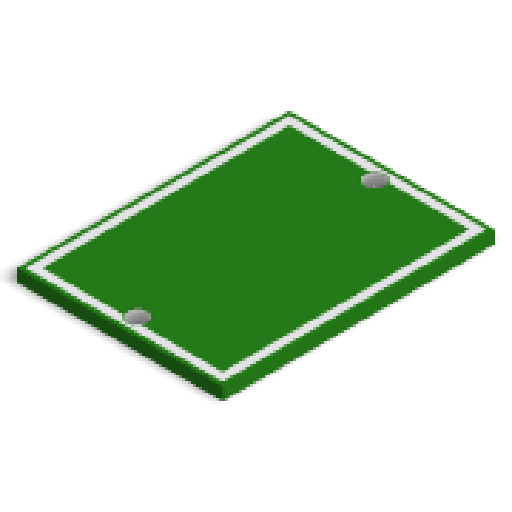
# Autodesk Inventor part: PIR sensor
Saved by Autodesk Inventor 2024 (Build 280153000, 153)
## iProperties
Created: 2024-09-23
Part Number: PIR sensor
Material: Generic
Document SubType Name: Modeling
Designer: Laith Al-Sadi
Density: 1 g/cm^3
Appearance: Default
Author: Laith Al-Sadi
Autodesk Inventor part; units mm, degrees
ref_plane "YZ Plane" through (0, 0, 0) normal (1, 0, 0) x (0, 1, 0)
ref_plane "XZ Plane" through (0, 0, 0) normal (0, 1, 0) x (-1, 0, 0)
ref_plane "XY Plane" through (0, 0, 0) normal (0, 0, 1) x (1, 0, 0)
sketch "Sketch1" plane through (0, 0, 0) normal (0, 1, 0) x (-1, 0, 0)
  line L0 (12.15, 16.1) -> (-12.15, 16.1)
  line L1 (-12.15, 16.1) -> (-12.15, -16.1)
  line L2 (-12.15, -16.1) -> (12.15, -16.1)
  line L3 (12.15, -16.1) -> (12.15, 16.1)
  line L4 (12.15, 16.1) -> (-12.15, -16.1) construction
  line L5 (-12.15, 16.1) -> (12.15, -16.1) construction
  circle A0 centre (0, 14) radius 1.15
  circle A1 centre (0, -14) radius 1.15
  point P0 (0, 0)
  dimension "d0" = 32.2
  dimension "d1" = 24.3
  dimension "d4" = 2.3
  dimension "d5" = 2.3
  dimension "d6" = 28
  dimension "d7" = 14
  constraints: 12 end point, 2 centre point, 2 midpoint, 2 parallel, 2 vertical alignment, 1 horizontal, 1 perpendicular
  measures "d0" distance of L2.end L0.start
  measures "d1" distance of L1.end L2.end
  measures "d4" diameter of A0
  measures "d5" diameter of A1
  measures "d6" distance of A1.centre A0.centre
  measures "d7" distance of point (0, 0) A0.centre
extrude "Extrusion1" add sketch "Sketch1" along normal blind 1.5
sketch "Sketch2" plane through (0, 1.5, 0) normal (0, 1, 0) x (1, 0, 0)
  line L0 (12.15, -16.1) -> (12.15, 16.1) projected
  line L1 (12.15, 16.1) -> (-12.15, 16.1) projected
  line L2 (-12.15, 16.1) -> (-12.15, -16.1) projected
  line L3 (-12.15, -16.1) -> (12.15, -16.1) projected
  circle A0 centre (0, -14) radius 1.15 projected
  circle A1 centre (0, 14) radius 1.15 projected
  line L4 (-11.65, -15.6) -> (-11.65, 15.6)
  line L5 (-11.65, 15.6) -> (11.65, 15.6)
  line L6 (11.65, 15.6) -> (11.65, -15.6)
  line L7 (11.65, -15.6) -> (-11.65, -15.6)
  line L8 (-10.65, 14.6) -> (-10.65, -14.6)
  line L9 (-10.65, -14.6) -> (10.65, -14.6)
  line L10 (10.65, -14.6) -> (10.65, 14.6)
  line L11 (10.65, 14.6) -> (-10.65, 14.6)
  point P0 (0, 0)
  point P1 (-0.9811, 14.6)
  point P2 (0.9811, 14.6)
  point P3 (0.9811, -14.6)
  point P4 (-0.9811, -14.6)
  dimension "d8" = 0.5
  dimension "d9" = 1
  constraints: 16 end point, 6 other
  measures "d8" distance between parallel lines of L2 L4
  measures "d9" distance between parallel lines of L4 L8
extrude "Extrusion2" add sketch "Sketch2" along normal blind 0.01 contours L4 L5 L6 L7
sketch "Sketch3" plane through (0, 1.5, 0) normal (0, 1, 0) x (1, 0, 0)
  circle A0 centre (0, -14) radius 1.15 projected
  circle A1 centre (0, -14) radius 1.2525
  arc A2 (-0.9811, 14.6) -> (0.9811, 14.6) centre (0, 14) ccw projected
  circle A3 centre (0, 14) radius 1.2525
  point P0 (0, 0)
  dimension "d12" = 2.505
  dimension "d13" = 2.505
  constraints: 2 centre point, 2 coincident
  measures "d12" diameter of A1
  measures "d13" diameter of A3
extrude "Extrusion3" cut sketch "Sketch3" along normal up to surface (0.01 mm away)
sketch "Sketch4" plane through (0, 0, 0) normal (0, -1, 0) x (1, 0, 0)
  line L0 (-11.45, 3) -> (-11.45, -3) construction
  line L1 (-11.45, -3) -> (-12.15, -3) construction
  line L2 (-12.15, -3) -> (-12.15, 3) construction
  line L3 (-12.15, 3) -> (-11.45, 3) construction
  line L4 (-12.15, -16.1) -> (-12.15, 16.1) projected
  line L5 (11.3793, -5.3256) -> (11.3793, 5.3256) construction
  line L6 (11.3793, 5.3256) -> (20.3774, 5.3256) construction
  line L7 (20.3774, 5.3256) -> (20.3774, -5.3256) construction
  line L8 (20.3774, -5.3256) -> (11.3793, -5.3256) construction
  line L9 (12.15, 16.1) -> (12.15, -16.1) projected
  spline S0 degree 2 poles (-11.6479, 2.8207) (-11.7346, 2.8207) (-11.8493, 2.7865) (-11.8493, 2.7444) knots 0 0 0 1 2 2 2
  spline S1 degree 2 poles (-11.8493, 2.7444) (-11.8493, 2.7237) (-11.8327, 2.7016) (-11.8127, 2.696) (-11.7851, 2.695) (-11.7647, 2.695) knots 0 0 0 1 2 3 4 4 4
  line L10 (-11.7647, 2.695) -> (-11.7433, 2.695)
  spline S2 degree 2 poles (-11.7433, 2.695) (-11.7198, 2.695) (-11.7115, 2.6967) knots 0 0 0 1 1 1
  spline S3 degree 2 poles (-11.7115, 2.6967) (-11.6935, 2.6981) (-11.6804, 2.7098) (-11.6769, 2.734) (-11.6766, 2.7537) (-11.6759, 2.762) knots 0 0 0 1 2 3 4 4 4
  line L11 (-11.6759, 2.762) -> (-11.6673, 2.762)
  line L12 (-11.6673, 2.762) -> (-11.6673, 2.505)
  line L13 (-11.6673, 2.505) -> (-11.6759, 2.505)
  line L14 (-11.6759, 2.505) -> (-11.6776, 2.5302)
  spline S4 degree 2 poles (-11.6776, 2.5302) (-11.6794, 2.5472) (-11.6918, 2.5585) (-11.7104, 2.5603) knots 0 0 0 1 2 2 2
  line L15 (-11.7104, 2.5603) -> (-11.7364, 2.5613)
  line L16 (-11.7364, 2.5613) -> (-11.8082, 2.5613)
  line L17 (-11.8082, 2.5613) -> (-11.8576, 2.5603)
  line L18 (-11.8576, 2.5603) -> (-11.8576, 2.5686)
  spline S5 degree 2 poles (-11.8576, 2.5686) (-11.8417, 2.5758) (-11.8151, 2.6114) (-11.8151, 2.6328) knots 0 0 0 1 2 2 2
  spline S6 degree 2 poles (-11.8151, 2.6328) (-11.8151, 2.6518) (-11.8624, 2.7233) (-11.8624, 2.782) knots 0 0 0 1 2 2 2
  spline S7 degree 2 poles (-11.8624, 2.782) (-11.8624, 2.8632) (-11.745, 2.9741) (-11.6562, 2.9741) knots 0 0 0 1 2 2 2
  spline S8 degree 2 poles (-11.6562, 2.9741) (-11.563, 2.9741) (-11.45, 2.8522) (-11.45, 2.7579) knots 0 0 0 1 2 2 2
  spline S9 degree 2 poles (-11.45, 2.7579) (-11.45, 2.7064) (-11.4959, 2.6142) (-11.497, 2.6086) knots 0 0 0 1 2 2 2
  spline S10 degree 2 poles (-11.497, 2.6086) (-11.497, 2.5927) (-11.4735, 2.5817) (-11.4514, 2.5769) knots 0 0 0 1 2 2 2
  line L19 (-11.4514, 2.5769) -> (-11.4514, 2.5658)
  line L20 (-11.4514, 2.5658) -> (-11.6286, 2.5658)
  line L21 (-11.6286, 2.5658) -> (-11.6286, 2.5751)
  spline S11 degree 2 poles (-11.6286, 2.5751) (-11.5609, 2.5917) (-11.4666, 2.668) (-11.4666, 2.7275) knots 0 0 0 1 2 2 2
  spline S12 degree 2 poles (-11.4666, 2.7275) (-11.4666, 2.7744) (-11.5757, 2.8207) (-11.6479, 2.8207) knots 0 0 0 1 2 2 2
  spline S13 degree 2 poles (-11.4645, 2.0093) (-11.4652, 2.0166) (-11.4662, 2.0335) (-11.4711, 2.0642) (-11.4915, 2.0801) (-11.5091, 2.0819) knots 0 0 0 1 2 3 4 4 4
  line L22 (-11.5091, 2.0819) -> (-11.5353, 2.0829)
  line L23 (-11.5353, 2.0829) -> (-11.8559, 2.0829)
  line L24 (-11.8559, 2.0829) -> (-11.8559, 2.1499)
  line L25 (-11.8559, 2.1499) -> (-11.5222, 2.4107)
  line L26 (-11.5222, 2.4107) -> (-11.5222, 2.4128)
  line L27 (-11.5222, 2.4128) -> (-11.7785, 2.4128)
  line L28 (-11.7785, 2.4128) -> (-11.8051, 2.4117)
  spline S14 degree 2 poles (-11.8051, 2.4117) (-11.8231, 2.41) (-11.8407, 2.3952) (-11.8455, 2.3651) (-11.8465, 2.3437) (-11.8472, 2.3399) knots 0 0 0 1 2 3 4 4 4
  line L29 (-11.8472, 2.3399) -> (-11.8559, 2.3399)
  line L30 (-11.8559, 2.3399) -> (-11.8559, 2.4981)
  line L31 (-11.8559, 2.4981) -> (-11.8472, 2.4981)
  spline S15 degree 2 poles (-11.8472, 2.4981) (-11.8465, 2.4908) (-11.8455, 2.4732) (-11.8386, 2.4287) (-11.8051, 2.4252) knots 0 0 0 1 2 3 3 3
  line L32 (-11.8051, 2.4252) -> (-11.7785, 2.4242)
  line L33 (-11.7785, 2.4242) -> (-11.5288, 2.4242)
  line L34 (-11.5288, 2.4242) -> (-11.5035, 2.4252)
  spline S16 degree 2 poles (-11.5035, 2.4252) (-11.4918, 2.4325) (-11.4721, 2.4522) (-11.4645, 2.476) (-11.4645, 2.487) knots 0 0 0 1 2 3 3 3
  line L35 (-11.4645, 2.487) -> (-11.4645, 2.5036)
  line L36 (-11.4645, 2.5036) -> (-11.4559, 2.5036)
  line L37 (-11.4559, 2.5036) -> (-11.4559, 2.2936)
  line L38 (-11.4559, 2.2936) -> (-11.7084, 2.0964)
  line L39 (-11.7084, 2.0964) -> (-11.7084, 2.0943)
  line L40 (-11.7084, 2.0943) -> (-11.5332, 2.0943)
  line L41 (-11.5332, 2.0943) -> (-11.507, 2.0953)
  spline S17 degree 2 poles (-11.507, 2.0953) (-11.4894, 2.0971) (-11.4711, 2.1119) (-11.4662, 2.1416) (-11.4652, 2.1596) (-11.4645, 2.1672) knots 0 0 0 1 2 3 4 4 4
  line L42 (-11.4645, 2.1672) -> (-11.4559, 2.1672)
  line L43 (-11.4559, 2.1672) -> (-11.4559, 2.0093)
  line L44 (-11.4559, 2.0093) -> (-11.4645, 2.0093)
  line L45 (-11.8559, 1.9921) -> (-11.8472, 1.9921)
  spline S18 degree 2 poles (-11.8472, 1.9921) (-11.8472, 1.9851) (-11.8455, 1.9665) (-11.8427, 1.9427) (-11.8293, 1.9302) (-11.8117, 1.9285) knots 0 0 0 1 2 3 4 4 4
  line L46 (-11.8117, 1.9285) -> (-11.7864, 1.9275)
  line L47 (-11.7864, 1.9275) -> (-11.526, 1.9275)
  line L48 (-11.526, 1.9275) -> (-11.5008, 1.9285)
  spline S19 degree 2 poles (-11.5008, 1.9285) (-11.4832, 1.9302) (-11.469, 1.9434) (-11.4655, 1.9668) (-11.4652, 1.9862) (-11.4645, 1.9938) knots 0 0 0 1 2 3 4 4 4
  line L49 (-11.4645, 1.9938) -> (-11.4559, 1.9938)
  line L50 (-11.4559, 1.9938) -> (-11.4545, 1.7893)
  spline S20 degree 2 poles (-11.4545, 1.7893) (-11.4545, 1.725) (-11.4787, 1.6114) (-11.5775, 1.5154) (-11.6676, 1.5154) knots 0 0 0 1 2 3 3 3
  spline S21 degree 2 poles (-11.6676, 1.5154) (-11.7536, 1.5154) (-11.8355, 1.6014) (-11.8559, 1.6974) (-11.8559, 1.7613) knots 0 0 0 1 2 3 3 3
  line L51 (-11.8559, 1.7613) -> (-11.8559, 1.9921)
  spline S22 degree 2 poles (-11.4718, 1.7344) (-11.4683, 1.7423) (-11.4662, 1.7744) (-11.4662, 1.7862) knots 0 0 0 1 2 2 2
  line L52 (-11.4662, 1.7862) -> (-11.4662, 1.7927)
  line L53 (-11.4662, 1.7927) -> (-11.8455, 1.7927)
  spline S23 degree 2 poles (-11.8455, 1.7927) (-11.8455, 1.7889) (-11.8462, 1.7824) (-11.8462, 1.7772) knots 0 0 0 1 2 2 2
  spline S24 degree 2 poles (-11.8462, 1.7772) (-11.8462, 1.7565) (-11.8407, 1.7219) (-11.8182, 1.6915) (-11.7212, 1.6636) (-11.67, 1.6636) knots 0 0 0 1 2 3 4 4 4
  spline S25 degree 2 poles (-11.67, 1.6636) (-11.5985, 1.6636) (-11.4859, 1.6981) (-11.4718, 1.7344) knots 0 0 0 1 2 2 2
  spline S26 degree 2 poles (-11.6562, 0.3344) (-11.744, 0.3344) (-11.8624, 0.4674) (-11.8624, 0.5579) knots 0 0 0 1 2 2 2
  spline S27 degree 2 poles (-11.8624, 0.5579) (-11.8624, 0.6522) (-11.7457, 0.7789) (-11.6562, 0.7789) knots 0 0 0 1 2 2 2
  spline S28 degree 2 poles (-11.6562, 0.7789) (-11.564, 0.7789) (-11.45, 0.6494) (-11.45, 0.5579) knots 0 0 0 1 2 2 2
  spline S29 degree 2 poles (-11.45, 0.5579) (-11.45, 0.466) (-11.5657, 0.3344) (-11.6562, 0.3344) knots 0 0 0 1 2 2 2
  spline S30 degree 2 poles (-11.5063, 0.5012) (-11.4604, 0.5174) (-11.4604, 0.5575) knots 0 0 0 1 1 1
  spline S31 degree 2 poles (-11.4604, 0.5575) (-11.4604, 0.5779) (-11.4866, 0.6076) (-11.5367, 0.6235) (-11.6151, 0.6307) (-11.6562, 0.6307) knots 0 0 0 1 2 3 4 4 4
  spline S32 degree 2 poles (-11.6562, 0.6307) (-11.7129, 0.6307) (-11.784, 0.6221) (-11.8521, 0.5979) (-11.8521, 0.5575) knots 0 0 0 1 2 3 3 3
  spline S33 degree 2 poles (-11.8521, 0.5575) (-11.8521, 0.5375) (-11.8258, 0.5078) (-11.7757, 0.4919) (-11.6973, 0.4846) (-11.6562, 0.4846) knots 0 0 0 1 2 3 4 4 4
  spline S34 degree 2 poles (-11.6562, 0.4846) (-11.6075, 0.4846) (-11.5357, 0.4912) (-11.5063, 0.5012) knots 0 0 0 1 2 2 2
  spline S35 degree 2 poles (-11.4645, -0.1689) (-11.4652, -0.1617) (-11.4662, -0.1434) (-11.4704, -0.1133) (-11.4925, -0.0974) (-11.5101, -0.0957) knots 0 0 0 1 2 3 4 4 4
  line L54 (-11.5101, -0.0957) -> (-11.5364, -0.0946)
  line L55 (-11.5364, -0.0946) -> (-11.6994, -0.0946)
  line L56 (-11.6994, -0.0946) -> (-11.727, -0.0936)
  spline S36 degree 2 poles (-11.727, -0.0936) (-11.8027, -0.0853) (-11.8624, -0.0193) (-11.8624, 0.0497) knots 0 0 0 1 2 2 2
  spline S37 degree 2 poles (-11.8624, 0.0497) (-11.8624, 0.1406) (-11.7934, 0.2394) (-11.7415, 0.2394) knots 0 0 0 1 2 2 2
  line L57 (-11.7415, 0.2394) -> (-11.5253, 0.2394)
  line L58 (-11.5253, 0.2394) -> (-11.5001, 0.2404)
  spline S38 degree 2 poles (-11.5001, 0.2404) (-11.4825, 0.2421) (-11.469, 0.2535) (-11.4666, 0.2708) knots 0 0 0 1 2 2 2
  line L59 (-11.4666, 0.2708) -> (-11.4645, 0.2936)
  line L60 (-11.4645, 0.2936) -> (-11.4559, 0.2936)
  line L61 (-11.4559, 0.2936) -> (-11.4559, 0.037)
  line L62 (-11.4559, 0.037) -> (-11.4645, 0.037)
  spline S39 degree 2 poles (-11.4645, 0.037) (-11.4652, 0.0442) (-11.4655, 0.0625) (-11.4693, 0.0908) (-11.4814, 0.1019) (-11.5001, 0.1036) knots 0 0 0 1 2 3 4 4 4
  line L63 (-11.5001, 0.1036) -> (-11.5256, 0.1047)
  line L64 (-11.5256, 0.1047) -> (-11.7457, 0.1047)
  spline S40 degree 2 poles (-11.7457, 0.1047) (-11.7522, 0.1047) (-11.7709, 0.1036) (-11.8099, 0.0974) (-11.8479, 0.0598) (-11.8479, 0.0266) knots 0 0 0 1 2 3 4 4 4
  spline S41 degree 2 poles (-11.8479, 0.0266) (-11.8479, -0.0193) (-11.8013, -0.0663) (-11.7408, -0.0822) (-11.7194, -0.0826) knots 0 0 0 1 2 3 3 3
  line L65 (-11.7194, -0.0826) -> (-11.6935, -0.0832)
  line L66 (-11.6935, -0.0832) -> (-11.5343, -0.0832)
  line L67 (-11.5343, -0.0832) -> (-11.508, -0.0822)
  spline S42 degree 2 poles (-11.508, -0.0822) (-11.4897, -0.0805) (-11.4711, -0.0656) (-11.4662, -0.0359) (-11.4652, -0.0162) (-11.4645, -0.0073) knots 0 0 0 1 2 3 4 4 4
  line L68 (-11.4645, -0.0073) -> (-11.4559, -0.0073)
  line L69 (-11.4559, -0.0073) -> (-11.4559, -0.1689)
  line L70 (-11.4559, -0.1689) -> (-11.4645, -0.1689)
  line L71 (-11.4559, -0.1634) -> (-11.4559, -0.5965)
  line L72 (-11.4559, -0.5965) -> (-11.632, -0.5965)
  line L73 (-11.632, -0.5965) -> (-11.632, -0.5872)
  spline S43 degree 2 poles (-11.632, -0.5872) (-11.5985, -0.5724) (-11.5232, -0.5313) (-11.4673, -0.4864) (-11.4673, -0.4694) knots 0 0 0 1 2 3 3 3
  line L74 (-11.4673, -0.4694) -> (-11.4662, -0.4473)
  line L75 (-11.4662, -0.4473) -> (-11.7864, -0.4473)
  line L76 (-11.7864, -0.4473) -> (-11.8117, -0.4484)
  spline S44 degree 2 poles (-11.8117, -0.4484) (-11.8293, -0.4501) (-11.8427, -0.4615) (-11.8455, -0.4857) (-11.8465, -0.5054) (-11.8472, -0.5133) knots 0 0 0 1 2 3 4 4 4
  line L77 (-11.8472, -0.5133) -> (-11.8559, -0.5133)
  line L78 (-11.8559, -0.5133) -> (-11.8559, -0.2453)
  line L79 (-11.8559, -0.2453) -> (-11.8472, -0.2453)
  line L80 (-11.8472, -0.2453) -> (-11.8455, -0.2812)
  spline S45 degree 2 poles (-11.8455, -0.2812) (-11.8438, -0.2978) (-11.8307, -0.3098) (-11.8127, -0.3116) knots 0 0 0 1 2 2 2
  line L81 (-11.8127, -0.3116) -> (-11.7875, -0.3126)
  line L82 (-11.7875, -0.3126) -> (-11.4662, -0.3126)
  line L83 (-11.4662, -0.3126) -> (-11.4673, -0.2912)
  spline S46 degree 2 poles (-11.4673, -0.2912) (-11.4673, -0.2736) (-11.5194, -0.2307) (-11.5992, -0.1876) (-11.632, -0.1727) knots 0 0 0 1 2 3 3 3
  line L84 (-11.632, -0.1727) -> (-11.632, -0.1634)
  line L85 (-11.632, -0.1634) -> (-11.4559, -0.1634)
  line L86 (-11.5125, -1.3993) -> (-11.6535, -1.3993)
  line L87 (-11.6535, -1.3993) -> (-11.6535, -1.5375)
  line L88 (-11.6535, -1.5375) -> (-11.698, -1.5375)
  line L89 (-11.698, -1.5375) -> (-11.698, -1.3993)
  line L90 (-11.698, -1.3993) -> (-11.8396, -1.3993)
  line L91 (-11.8396, -1.3993) -> (-11.8396, -1.3547)
  line L92 (-11.8396, -1.3547) -> (-11.698, -1.3547)
  line L93 (-11.698, -1.3547) -> (-11.698, -1.2166)
  line L94 (-11.698, -1.2166) -> (-11.6535, -1.2166)
  line L95 (-11.6535, -1.2166) -> (-11.6535, -1.3547)
  line L96 (-11.6535, -1.3547) -> (-11.5125, -1.3547)
  line L97 (-11.5125, -1.3547) -> (-11.5125, -1.3993)
  line L98 (-11.6693, -1.6477) -> (-11.4524, -1.6953)
  line L99 (-11.4524, -1.6953) -> (-11.4524, -1.7002)
  spline S47 degree 2 poles (-11.4524, -1.7002) (-11.4586, -1.7195) (-11.4707, -1.7737) (-11.4707, -1.8069) knots 0 0 0 1 2 2 2
  spline S48 degree 2 poles (-11.4707, -1.8069) (-11.4707, -1.849) (-11.4645, -1.8756) knots 0 0 0 1 1 1
  spline S49 degree 2 poles (-11.4645, -1.8756) (-11.4579, -1.8933) (-11.4507, -1.9109) knots 0 0 0 1 1 1
  spline S50 degree 2 poles (-11.4507, -1.9109) (-11.4507, -1.9161) (-11.4611, -1.9161) knots 0 0 0 1 1 1
  spline S51 degree 2 poles (-11.4611, -1.9161) (-11.4776, -1.9161) (-11.5201, -1.8915) (-11.5668, -1.8318) (-11.5668, -1.7689) knots 0 0 0 1 2 3 3 3
  spline S52 degree 2 poles (-11.5668, -1.7689) (-11.5668, -1.7409) (-11.5609, -1.7016) (-11.5526, -1.6839) knots 0 0 0 1 2 2 2
  line L100 (-11.5526, -1.6839) -> (-11.6296, -1.6663)
  spline S53 degree 2 poles (-11.6296, -1.6663) (-11.6051, -1.6915) (-11.5871, -1.7527) (-11.5871, -1.8007) knots 0 0 0 1 2 2 2
  spline S54 degree 2 poles (-11.5871, -1.8007) (-11.5871, -1.8618) (-11.6573, -1.9551) (-11.7139, -1.9551) knots 0 0 0 1 2 2 2
  spline S55 degree 2 poles (-11.7139, -1.9551) (-11.7847, -1.9551) (-11.8624, -1.8339) (-11.8624, -1.7544) knots 0 0 0 1 2 2 2
  spline S56 degree 2 poles (-11.8624, -1.7544) (-11.8624, -1.694) (-11.8047, -1.6176) (-11.7609, -1.6176) knots 0 0 0 1 2 2 2
  spline S57 degree 2 poles (-11.7609, -1.6176) (-11.7381, -1.6176) (-11.7039, -1.6549) (-11.7039, -1.6798) knots 0 0 0 1 2 2 2
  spline S58 degree 2 poles (-11.7039, -1.6798) (-11.7039, -1.7098) (-11.7364, -1.7516) (-11.7636, -1.7516) knots 0 0 0 1 2 2 2
  spline S59 degree 2 poles (-11.7636, -1.7516) (-11.7913, -1.7516) (-11.8265, -1.7164) (-11.8334, -1.7164) knots 0 0 0 1 2 2 2
  spline S60 degree 2 poles (-11.8334, -1.7164) (-11.8434, -1.7164) (-11.8538, -1.7399) (-11.8538, -1.752) knots 0 0 0 1 2 2 2
  spline S61 degree 2 poles (-11.8538, -1.752) (-11.8538, -1.7934) (-11.7868, -1.8231) (-11.7367, -1.8231) knots 0 0 0 1 2 2 2
  spline S62 degree 2 poles (-11.7367, -1.8231) (-11.6835, -1.8231) (-11.6023, -1.7862) (-11.6023, -1.7444) knots 0 0 0 1 2 2 2
  spline S63 degree 2 poles (-11.6023, -1.7444) (-11.6023, -1.7064) (-11.6396, -1.6691) (-11.6593, -1.6587) (-11.6704, -1.656) knots 0 0 0 1 2 3 3 3
  line L101 (-11.6704, -1.656) -> (-11.6693, -1.6477)
  spline S64 degree 2 poles (-11.4645, -2.4104) (-11.4652, -2.4055) (-11.4655, -2.3924) (-11.47, -2.3644) (-11.4842, -2.3444) (-11.5025, -2.3368) knots 0 0 0 1 2 3 4 4 4
  line L102 (-11.5025, -2.3368) -> (-11.5446, -2.3202)
  line L103 (-11.5446, -2.3202) -> (-11.8579, -2.21)
  line L104 (-11.8579, -2.21) -> (-11.8579, -2.1534)
  line L105 (-11.8579, -2.1534) -> (-11.5436, -2.0415)
  line L106 (-11.5436, -2.0415) -> (-11.5008, -2.0245)
  spline S65 degree 2 poles (-11.5008, -2.0245) (-11.4832, -2.0162) (-11.4683, -2.0007) (-11.4666, -1.9865) knots 0 0 0 1 2 2 2
  line L107 (-11.4666, -1.9865) -> (-11.4645, -1.9641)
  line L108 (-11.4645, -1.9641) -> (-11.4559, -1.9641)
  line L109 (-11.4559, -1.9641) -> (-11.4559, -2.218)
  line L110 (-11.4559, -2.218) -> (-11.4645, -2.218)
  line L111 (-11.4645, -2.218) -> (-11.4666, -2.1938)
  spline S66 degree 2 poles (-11.4666, -2.1938) (-11.469, -2.1817) (-11.4745, -2.1668) (-11.4887, -2.1668) knots 0 0 0 1 2 2 2
  spline S67 degree 2 poles (-11.4887, -2.1668) (-11.4984, -2.1668) (-11.5467, -2.1827) (-11.6331, -2.2145) (-11.717, -2.2466) knots 0 0 0 1 2 3 3 3
  spline S68 degree 2 poles (-11.717, -2.2466) (-11.6652, -2.2656) (-11.555, -2.3054) (-11.5063, -2.3195) (-11.4942, -2.3195) knots 0 0 0 1 2 3 3 3
  spline S69 degree 2 poles (-11.4942, -2.3195) (-11.4804, -2.3195) (-11.4693, -2.3064) (-11.4655, -2.2888) (-11.4652, -2.2718) (-11.4645, -2.2646) knots 0 0 0 1 2 3 4 4 4
  line L112 (-11.4645, -2.2646) -> (-11.4559, -2.2646)
  line L113 (-11.4559, -2.2646) -> (-11.4559, -2.4104)
  line L114 (-11.4559, -2.4104) -> (-11.4645, -2.4104)
  spline S70 degree 2 poles (11.8971, -5.1356) (11.8971, -5.1899) (11.8744, -5.266) (11.8582, -5.2997) knots 0 0 0 1 2 2 2
  line L115 (11.8582, -5.2997) -> (11.7747, -5.2997)
  line L116 (11.7747, -5.2997) -> (11.7747, -5.2948)
  spline S71 degree 2 poles (11.7747, -5.2948) (11.8055, -5.262) (11.8395, -5.1789) (11.8395, -5.1404) knots 0 0 0 1 2 2 2
  spline S72 degree 2 poles (11.8395, -5.1404) (11.8395, -5.0853) (11.7938, -5.029) (11.7561, -5.029) knots 0 0 0 1 2 2 2
  spline S73 degree 2 poles (11.7561, -5.029) (11.7261, -5.029) (11.6888, -5.0586) (11.6795, -5.0906) knots 0 0 0 1 2 2 2
  spline S74 degree 2 poles (11.6795, -5.0906) (11.673, -5.1137) (11.6641, -5.1522) (11.6568, -5.1809) knots 0 0 0 1 2 2 2
  spline S75 degree 2 poles (11.6568, -5.1809) (11.6499, -5.2069) (11.6293, -5.2478) (11.6126, -5.2636) knots 0 0 0 1 2 2 2
  spline S76 degree 2 poles (11.6126, -5.2636) (11.596, -5.279) (11.5515, -5.296) (11.5223, -5.296) knots 0 0 0 1 2 2 2
  spline S77 degree 2 poles (11.5223, -5.296) (11.4615, -5.296) (11.3793, -5.2012) (11.3793, -5.1279) knots 0 0 0 1 2 2 2
  spline S78 degree 2 poles (11.3793, -5.1279) (11.3793, -5.0857) (11.3959, -5.0112) (11.4117, -4.9792) knots 0 0 0 1 2 2 2
  line L117 (11.4117, -4.9792) -> (11.4911, -4.9792)
  line L118 (11.4911, -4.9792) -> (11.4911, -4.984)
  spline S79 degree 2 poles (11.4911, -4.984) (11.4692, -5.0079) (11.4368, -5.0825) (11.4368, -5.1234) knots 0 0 0 1 2 2 2
  spline S80 degree 2 poles (11.4368, -5.1234) (11.4368, -5.1696) (11.4801, -5.2267) (11.5154, -5.2267) knots 0 0 0 1 2 2 2
  spline S81 degree 2 poles (11.5154, -5.2267) (11.547, -5.2267) (11.5847, -5.1931) (11.5932, -5.1615) knots 0 0 0 1 2 2 2
  spline S82 degree 2 poles (11.5932, -5.1615) (11.5989, -5.1404) (11.6135, -5.0792) (11.6195, -5.059) knots 0 0 0 1 2 2 2
  spline S83 degree 2 poles (11.6195, -5.059) (11.6353, -5.0075) (11.6989, -4.9597) (11.7455, -4.9597) knots 0 0 0 1 2 2 2
  spline S84 degree 2 poles (11.7455, -4.9597) (11.7751, -4.9597) (11.8319, -4.9836) (11.8517, -5.0051) knots 0 0 0 1 2 2 2
  spline S85 degree 2 poles (11.8517, -5.0051) (11.8736, -5.029) (11.8971, -5.0898) (11.8971, -5.1356) knots 0 0 0 1 2 2 2
  line L119 (11.8882, -4.892) -> (11.3882, -4.892)
  line L120 (11.3882, -4.892) -> (11.3882, -4.5792)
  line L121 (11.3882, -4.5792) -> (11.4473, -4.5792)
  line L122 (11.4473, -4.5792) -> (11.4473, -4.8256)
  line L123 (11.4473, -4.8256) -> (11.5843, -4.8256)
  line L124 (11.5843, -4.8256) -> (11.5843, -4.5959)
  line L125 (11.5843, -4.5959) -> (11.6434, -4.5959)
  line L126 (11.6434, -4.5959) -> (11.6434, -4.8256)
  line L127 (11.6434, -4.8256) -> (11.829, -4.8256)
  line L128 (11.829, -4.8256) -> (11.829, -4.5792)
  line L129 (11.829, -4.5792) -> (11.8882, -4.5792)
  line L130 (11.8882, -4.5792) -> (11.8882, -4.892)
  line L131 (11.8882, -4.1485) -> (11.8882, -4.2231)
  line L132 (11.8882, -4.2231) -> (11.4571, -4.4443)
  line L133 (11.4571, -4.4443) -> (11.8882, -4.4443)
  line L134 (11.8882, -4.4443) -> (11.8882, -4.5063)
  line L135 (11.8882, -4.5063) -> (11.3882, -4.5063)
  line L136 (11.3882, -4.5063) -> (11.3882, -4.4119)
  line L137 (11.3882, -4.4119) -> (11.784, -4.2105)
  line L138 (11.784, -4.2105) -> (11.3882, -4.2105)
  line L139 (11.3882, -4.2105) -> (11.3882, -4.1485)
  line L140 (11.3882, -4.1485) -> (11.8882, -4.1485)
  spline S86 degree 2 poles (11.8971, -3.9078) (11.8971, -3.9621) (11.8744, -4.0383) (11.8582, -4.0719) knots 0 0 0 1 2 2 2
  line L141 (11.8582, -4.0719) -> (11.7747, -4.0719)
  line L142 (11.7747, -4.0719) -> (11.7747, -4.0671)
  spline S87 degree 2 poles (11.7747, -4.0671) (11.8055, -4.0343) (11.8395, -3.9512) (11.8395, -3.9127) knots 0 0 0 1 2 2 2
  spline S88 degree 2 poles (11.8395, -3.9127) (11.8395, -3.8576) (11.7938, -3.8013) (11.7561, -3.8013) knots 0 0 0 1 2 2 2
  spline S89 degree 2 poles (11.7561, -3.8013) (11.7261, -3.8013) (11.6888, -3.8309) (11.6795, -3.8629) knots 0 0 0 1 2 2 2
  spline S90 degree 2 poles (11.6795, -3.8629) (11.673, -3.886) (11.6641, -3.9245) (11.6568, -3.9532) knots 0 0 0 1 2 2 2
  spline S91 degree 2 poles (11.6568, -3.9532) (11.6499, -3.9792) (11.6293, -4.0201) (11.6126, -4.0359) knots 0 0 0 1 2 2 2
  spline S92 degree 2 poles (11.6126, -4.0359) (11.596, -4.0513) (11.5515, -4.0683) (11.5223, -4.0683) knots 0 0 0 1 2 2 2
  spline S93 degree 2 poles (11.5223, -4.0683) (11.4615, -4.0683) (11.3793, -3.9735) (11.3793, -3.9001) knots 0 0 0 1 2 2 2
  spline S94 degree 2 poles (11.3793, -3.9001) (11.3793, -3.858) (11.3959, -3.7835) (11.4117, -3.7514) knots 0 0 0 1 2 2 2
  line L143 (11.4117, -3.7514) -> (11.4911, -3.7514)
  line L144 (11.4911, -3.7514) -> (11.4911, -3.7563)
  spline S95 degree 2 poles (11.4911, -3.7563) (11.4692, -3.7802) (11.4368, -3.8548) (11.4368, -3.8957) knots 0 0 0 1 2 2 2
  spline S96 degree 2 poles (11.4368, -3.8957) (11.4368, -3.9419) (11.4801, -3.999) (11.5154, -3.999) knots 0 0 0 1 2 2 2
  spline S97 degree 2 poles (11.5154, -3.999) (11.547, -3.999) (11.5847, -3.9654) (11.5932, -3.9338) knots 0 0 0 1 2 2 2
  spline S98 degree 2 poles (11.5932, -3.9338) (11.5989, -3.9127) (11.6135, -3.8515) (11.6195, -3.8313) knots 0 0 0 1 2 2 2
  spline S99 degree 2 poles (11.6195, -3.8313) (11.6353, -3.7798) (11.6989, -3.732) (11.7455, -3.732) knots 0 0 0 1 2 2 2
  spline S100 degree 2 poles (11.7455, -3.732) (11.7751, -3.732) (11.8319, -3.7559) (11.8517, -3.7774) knots 0 0 0 1 2 2 2
  spline S101 degree 2 poles (11.8517, -3.7774) (11.8736, -3.8013) (11.8971, -3.8621) (11.8971, -3.9078) knots 0 0 0 1 2 2 2
  line L145 (11.8882, -3.4901) -> (11.8882, -3.6838)
  line L146 (11.8882, -3.6838) -> (11.8371, -3.6838)
  line L147 (11.8371, -3.6838) -> (11.8371, -3.6202)
  line L148 (11.8371, -3.6202) -> (11.4392, -3.6202)
  line L149 (11.4392, -3.6202) -> (11.4392, -3.6838)
  line L150 (11.4392, -3.6838) -> (11.3882, -3.6838)
  line L151 (11.3882, -3.6838) -> (11.3882, -3.4901)
  line L152 (11.3882, -3.4901) -> (11.4392, -3.4901)
  line L153 (11.4392, -3.4901) -> (11.4392, -3.5537)
  line L154 (11.4392, -3.5537) -> (11.8371, -3.5537)
  line L155 (11.8371, -3.5537) -> (11.8371, -3.4901)
  line L156 (11.8371, -3.4901) -> (11.8882, -3.4901)
  line L157 (11.8882, -3.2911) -> (11.4473, -3.2911)
  line L158 (11.4473, -3.2911) -> (11.4473, -3.4589)
  line L159 (11.4473, -3.4589) -> (11.3882, -3.4589)
  line L160 (11.3882, -3.4589) -> (11.3882, -3.057)
  line L161 (11.3882, -3.057) -> (11.4473, -3.057)
  line L162 (11.4473, -3.057) -> (11.4473, -3.2247)
  line L163 (11.4473, -3.2247) -> (11.8882, -3.2247)
  line L164 (11.8882, -3.2247) -> (11.8882, -3.2911)
  line L165 (11.8882, -2.8321) -> (11.8882, -3.0258)
  line L166 (11.8882, -3.0258) -> (11.8371, -3.0258)
  line L167 (11.8371, -3.0258) -> (11.8371, -2.9621)
  line L168 (11.8371, -2.9621) -> (11.4392, -2.9621)
  line L169 (11.4392, -2.9621) -> (11.4392, -3.0258)
  line L170 (11.4392, -3.0258) -> (11.3882, -3.0258)
  line L171 (11.3882, -3.0258) -> (11.3882, -2.8321)
  line L172 (11.3882, -2.8321) -> (11.4392, -2.8321)
  line L173 (11.4392, -2.8321) -> (11.4392, -2.8957)
  line L174 (11.4392, -2.8957) -> (11.8371, -2.8957)
  line L175 (11.8371, -2.8957) -> (11.8371, -2.8321)
  line L176 (11.8371, -2.8321) -> (11.8882, -2.8321)
  line L177 (11.3882, -2.3872) -> (11.8882, -2.5594)
  line L178 (11.8882, -2.5594) -> (11.8882, -2.6311)
  line L179 (11.8882, -2.6311) -> (11.3882, -2.8033)
  line L180 (11.3882, -2.8033) -> (11.3882, -2.732)
  line L181 (11.3882, -2.732) -> (11.8035, -2.5934)
  line L182 (11.8035, -2.5934) -> (11.3882, -2.4548)
  line L183 (11.3882, -2.4548) -> (11.3882, -2.3872)
  line L184 (11.8882, -2.3394) -> (11.3882, -2.3394)
  line L185 (11.3882, -2.3394) -> (11.3882, -2.0266)
  line L186 (11.3882, -2.0266) -> (11.4473, -2.0266)
  line L187 (11.4473, -2.0266) -> (11.4473, -2.2729)
  line L188 (11.4473, -2.2729) -> (11.5843, -2.2729)
  line L189 (11.5843, -2.2729) -> (11.5843, -2.0432)
  line L190 (11.5843, -2.0432) -> (11.6434, -2.0432)
  line L191 (11.6434, -2.0432) -> (11.6434, -2.2729)
  line L192 (11.6434, -2.2729) -> (11.829, -2.2729)
  line L193 (11.829, -2.2729) -> (11.829, -2.0266)
  line L194 (11.829, -2.0266) -> (11.8882, -2.0266)
  line L195 (11.8882, -2.0266) -> (11.8882, -2.3394)
  line L196 (11.8882, 3.7465) -> (11.4473, 3.7465)
  line L197 (11.4473, 3.7465) -> (11.4473, 3.5788)
  line L198 (11.4473, 3.5788) -> (11.3882, 3.5788)
  line L199 (11.3882, 3.5788) -> (11.3882, 3.9807)
  line L200 (11.3882, 3.9807) -> (11.4473, 3.9807)
  line L201 (11.4473, 3.9807) -> (11.4473, 3.813)
  line L202 (11.4473, 3.813) -> (11.8882, 3.813)
  line L203 (11.8882, 3.813) -> (11.8882, 3.7465)
  line L204 (11.8882, 4.2056) -> (11.8882, 4.0119)
  line L205 (11.8882, 4.0119) -> (11.8371, 4.0119)
  line L206 (11.8371, 4.0119) -> (11.8371, 4.0755)
  line L207 (11.8371, 4.0755) -> (11.4392, 4.0755)
  line L208 (11.4392, 4.0755) -> (11.4392, 4.0119)
  line L209 (11.4392, 4.0119) -> (11.3882, 4.0119)
  line L210 (11.3882, 4.0119) -> (11.3882, 4.2056)
  line L211 (11.3882, 4.2056) -> (11.4392, 4.2056)
  line L212 (11.4392, 4.2056) -> (11.4392, 4.142)
  line L213 (11.4392, 4.142) -> (11.8371, 4.142)
  line L214 (11.8371, 4.142) -> (11.8371, 4.2056)
  line L215 (11.8371, 4.2056) -> (11.8882, 4.2056)
  line L216 (11.8882, 4.7165) -> (11.8882, 4.6501)
  line L217 (11.8882, 4.6501) -> (11.4575, 4.6501)
  line L218 (11.4575, 4.6501) -> (11.7504, 4.5196)
  line L219 (11.7504, 4.5196) -> (11.7504, 4.4791)
  line L220 (11.7504, 4.4791) -> (11.4575, 4.3499)
  line L221 (11.4575, 4.3499) -> (11.8882, 4.3499)
  line L222 (11.8882, 4.3499) -> (11.8882, 4.2879)
  line L223 (11.8882, 4.2879) -> (11.3882, 4.2879)
  line L224 (11.3882, 4.2879) -> (11.3882, 4.3786)
  line L225 (11.3882, 4.3786) -> (11.6665, 4.5034)
  line L226 (11.6665, 4.5034) -> (11.3882, 4.6242)
  line L227 (11.3882, 4.6242) -> (11.3882, 4.7165)
  line L228 (11.3882, 4.7165) -> (11.8882, 4.7165)
  line L229 (11.8882, 4.8178) -> (11.3882, 4.8178)
  line L230 (11.3882, 4.8178) -> (11.3882, 5.1306)
  line L231 (11.3882, 5.1306) -> (11.4473, 5.1306)
  line L232 (11.4473, 5.1306) -> (11.4473, 4.8843)
  line L233 (11.4473, 4.8843) -> (11.5843, 4.8843)
  line L234 (11.5843, 4.8843) -> (11.5843, 5.114)
  line L235 (11.5843, 5.114) -> (11.6434, 5.114)
  line L236 (11.6434, 5.114) -> (11.6434, 4.8843)
  line L237 (11.6434, 4.8843) -> (11.829, 4.8843)
  line L238 (11.829, 4.8843) -> (11.829, 5.1306)
  line L239 (11.829, 5.1306) -> (11.8882, 5.1306)
  line L240 (11.8882, 5.1306) -> (11.8882, 4.8178)
  point P0 (0, 0)
  point P1 (-11.45, 0)
  point P2 (-12.15, 0)
  point P3 (11.3793, 0)
  point P4 (12.15, 0)
  dimension "d16" = 0.7
  dimension "d17" = 0.7
  dimension "d18" = 6
  dimension "d21" = 8.9982
  dimension "d22" = 10.6512
  dimension "d23" = 0.7707
  constraints: 4 midpoint, 2 horizontal alignment, 2 vertical, 4 other
  measures "d16" distance from line of L4 point (-11.45, 0)
  measures "d17" distance of L0.end L1.end
  measures "d18" distance of L0.start L0.end
  measures "d21" distance of L5.end L6.end
  measures "d22" distance of L5.start L5.end
  measures "d23" distance between parallel lines of L9 L5
extrude "Extrusion4" cut sketch "Sketch4" against normal blind 0.1
equation "\"d7\" = 0.5 * d6"
body "Solid1"
